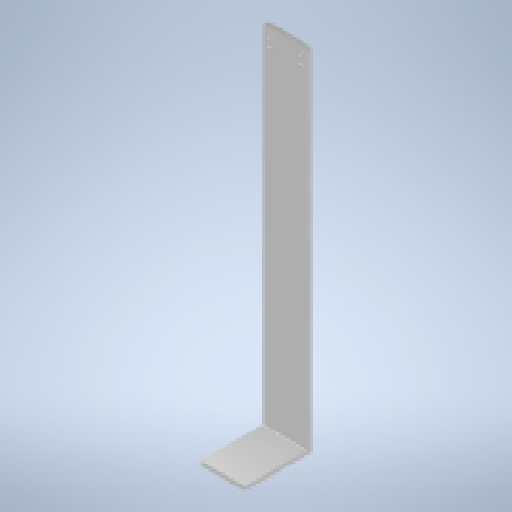
# Autodesk Inventor part: Bracket Holder
Saved by Autodesk Inventor 2025.3 (Build 293356000, 356)
## iProperties
Created: 2025-10-13
Part Number: Bracket Holder
Material: Aluminum 6061
Document SubType Name: Modeling
Designer: Haggag
Density: 2.7 g/cm^3
Appearance: Aluminum - Flat
Author: Haggag
Autodesk Inventor part; units mm, degrees
ref_plane "YZ Plane" through (0, 0, 0) normal (1, 0, 0) x (0, 1, 0)
ref_plane "XZ Plane" through (0, 0, 0) normal (0, 1, 0) x (-1, 0, 0)
ref_plane "XY Plane" through (0, 0, 0) normal (0, 0, 1) x (1, 0, 0)
sketch "Sketch2" plane through (0, 0, 0) normal (0, 0, 1) x (1, 0, 0)
  line L0 (-9.4794, 5.5186) -> (11.8294, 5.5186)
  circle A0 centre (-6.0645, -2.4947) radius 1.1
  circle A1 centre (8.4145, -2.4947) radius 1.1
  circle A2 centre (8.4145, 1.6737) radius 1.1
  circle A3 centre (-6.0645, 1.6737) radius 1.1
  line L1 (-9.4794, 5.5186) -> (-9.4794, -157.7914)
  line L2 (11.8294, -157.7914) -> (11.8294, 5.5186)
  line L3 (-9.4794, -157.7914) -> (-9.4794, -161.9314)
  line L4 (-9.4794, -161.9314) -> (11.8294, -161.9314)
  line L5 (11.8294, -161.9314) -> (11.8294, -157.7914)
  point P0 (0, 0)
  dimension "d20" = 163.31
  dimension "d31" = 4.14
  constraints: 12 end point, 4 centre point, 2 perpendicular, 2 vertical
  measures "d20" distance of L0.start L1.end
  measures "d31" distance of L1.end L3.end
extrude "Extrusion1" add sketch "Sketch2" along normal blind 2
fillet "Fillet6" radius 0.5 2 edges at (11.8294, 5.5186, 1) (-9.4794, 5.5186, 1)
sketch "Sketch9" plane through (0, 0, 2) normal (0, 0, 1) x (1, 0, 0)
  line L0 (-9.4794, -161.9314) -> (11.8294, -161.9314) projected
  line L1 (-9.4794, -161.9314) -> (11.8294, -161.9314)
  line L2 (11.8294, -161.9314) -> (11.8294, -159.9314)
  line L3 (11.8294, -159.9314) -> (-9.4794, -159.9314)
  line L4 (-9.4794, -159.9314) -> (-9.4794, -161.9314)
  point P0 (0, 0)
  dimension "d32" = 2
  constraints: 8 end point, 3 perpendicular, 1 collinear
  measures "d32" distance of L0.end L2.end
extrude "Extrusion7" add sketch "Sketch9" along normal blind 30
sketch "Sketch10" plane through (-9.4794, -159.9314, 2) normal (0, 1, 0) x (1, 0, 0)
  point P0 (9.4794, 2)
fillet "Fillet10" radius 0.5 2 edges at (1.175, -159.9314, 2) (1.175, -161.9314, 0)
fillet "Fillet11" radius 0.5 2 edges at (-9.4794, -160.9314, 32) (11.8294, -160.9314, 32)
body "Solid1"
